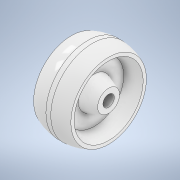
# Autodesk Inventor part: casterwheel
Saved by Autodesk Inventor 2020.3 (Build 243373000, 373)
## iProperties
Created: 2022-06-23
Part Number: casterwheel
Material: Nylon, molybdenum disulphide
Document SubType Name: Modeling
Designer: 0x6f736f646f
Density: 1.13 g/cm^3
Appearance: White
Author: 0x6f736f646f
Autodesk Inventor part; units mm, degrees
ref_plane "YZ Plane" through (0, 0, 0) normal (1, 0, 0) x (0, 1, 0)
ref_plane "XZ Plane" through (0, 0, 0) normal (0, 1, 0) x (-1, 0, 0)
ref_plane "XY Plane" through (0, 0, 0) normal (0, 0, 1) x (1, 0, 0)
sketch "Sketch1" plane through (0, 0, 0) normal (0, 1, 0) x (-1, 0, 0)
  line L0 (0, 0) -> (8.5, 0)
  line L1 (8.5, 0) -> (8.5, 19)
  line L2 (8.5, 19) -> (0, 19)
  line L3 (0, 19) -> (0, 0)
  line L4 (0, 2.6) -> (8.5, 2.6)
  line L5 (8.5, 5) -> (0, 5)
  line L6 (8.5, 5) -> (2, 7.3658)
  line L7 (2, 7.3658) -> (2, 13.3658)
  line L8 (2, 13.3658) -> (8.5, 15.7316)
  line L9 (8.5, 15.7316) -> (8.5, 17.2316)
  arc A0 (8.5, 17.2316) -> (0, 19) centre (0.5536, 0.3487) ccw
  line L10 (0, 0) -> (0, 28.973)
  line L11 (0, 0) -> (-8.5, 0)
  line L12 (-8.5, 0) -> (-8.5, 19)
  line L13 (-8.5, 19) -> (0, 19)
  line L14 (0, 2.6) -> (-8.5, 2.6)
  line L15 (-8.5, 5) -> (0, 5)
  line L16 (-8.5, 5) -> (-2, 7.3658)
  line L17 (-2, 7.3658) -> (-2, 13.3658)
  line L18 (-2, 13.3658) -> (-8.5, 15.7316)
  arc A1 (0, 19) -> (-8.5, 17.2316) centre (-0.5536, 0.3487) ccw
  line L19 (12.046, 0) -> (-12.046, 0) projected
  point P0 (1.1073, 19)
  point P1 (-1.1073, 19)
  dimension "d0" = 8.5
  dimension "d1" = 19
  dimension "d2" = 2.6
  dimension "d3" = 5
  dimension "d4" = 110
  dimension "d5" = 110
  dimension "d6" = 2
  dimension "d7" = 6
  dimension "d8" = 1.5
  dimension "d9" = 18.6595
  constraints: 38 end point, 10 point on line, 9 symmetric about line, 4 point on circle, 3 perpendicular, 2 centre point, 2 parallel, 2 vertical, 1 horizontal, 1 other
  measures "d0" distance of L2.end L1.end
  measures "d1" distance of L1.end L0.end
  measures "d2" distance between parallel lines of L0 L4
  measures "d3" distance between parallel lines of L0 L5
  measures "d4" angle of L7 L6
  measures "d5" angle of L7 L8
  measures "d6" distance between parallel lines of L3 L7
  measures "d7" distance of L6.end L7.end
  measures "d8" distance of L8.end L9.end
  measures "d9" radius of A0
revolve "Revolution1" add sketch "Sketch1" angle 360 about axis through (-10, 0, 0) along (1, 0, 0) contours L14 L12 L15 L3 | L3 L5 L1 L4 | L15 L16 L17 L18 L12 A1 L13 L3 | L3 L2 A0 L1 L8 L7 L6 L5
body "Solid1"
